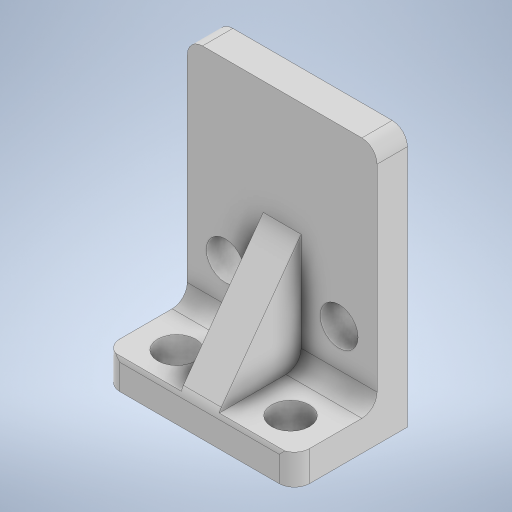
# Autodesk Inventor part: BP_L
Saved by Autodesk Inventor 2024.3 (Build 283343000, 343)
## iProperties
Created: 2025-10-31
Part Number: BP_L
Material: 一般
Document SubType Name: Modeling
Designer: 佐藤智貴
Density: 1 g/cm^3
Appearance: 既定
Author: 佐藤智貴
Autodesk Inventor part; units mm, degrees
ref_plane "YZ Plane" through (0, 0, 0) normal (1, 0, 0) x (0, 1, 0)
ref_plane "XZ Plane" through (0, 0, 0) normal (0, 1, 0) x (-1, 0, 0)
ref_plane "XY Plane" through (0, 0, 0) normal (0, 0, 1) x (1, 0, 0)
sketch "スケッチ1" plane through (0, 0, 0) normal (0, 0, 1) x (1, 0, 0)
  line L0 (0, 0) -> (25, 0)
  line L1 (25, 0) -> (25, 4)
  line L2 (25, 4) -> (0, 4)
  line L3 (0, 4) -> (0, 0)
  dimension "d0" = 4
  dimension "d1" = 25
  constraints: 8 end point, 2 parallel, 1 horizontal, 1 perpendicular
  measures "d0" distance of L0.end L1.end
  measures "d1" distance between parallel lines of L3 L1
extrude "押し出し1" add sketch "スケッチ1" along normal blind 18.9
sketch "スケッチ2" plane through (0, 4, 0) normal (0, 1, 0) x (1, 0, 0)
  line L0 (0, 0) -> (0, -18.9) projected
  line L1 (25, 0) -> (25, -18.9) projected
  line L2 (0, 0) -> (25, 0)
  line L3 (25, 0) -> (25, -8)
  line L4 (25, -8) -> (0, -8)
  line L5 (0, -8) -> (0, 0)
  point P0 (0, -8)
  dimension "d4" = 8
  constraints: 8 end point, 2 parallel, 1 horizontal, 1 perpendicular, 1 point on line
  measures "d4" distance between parallel lines of L2 L4
extrude "押し出し2" add sketch "スケッチ2" along normal blind 30
sketch "スケッチ3" plane through (0, 4, 18.9) normal (0, 1, 0) x (1, 0, 0)
  line L0 (0, 10.9) -> (25, 10.9) projected
  line L1 (25, 10.9) -> (25, 0) projected
  point P0 (0, 18.9)
  point P1 (5, 4.5)
  point P2 (20, 4.5)
  dimension "d7" = 15
  dimension "d8" = 6.4
  dimension "d9" = 6.4
  dimension "d10" = 5
  measures "d7" distance of point (20, 4.5) point (5, 4.5)
  measures "d8" distance from line of L0 point (5, 4.5)
  measures "d9" distance from line of L0 point (20, 4.5)
  measures "d10" distance from line of L1 point (20, 4.5)
hole "穴1" at (5, 4, 14.4) at (20, 4, 14.4) direction (0, -1, 0) diameter 5 end through all
sketch "スケッチ4" plane through (0, 4, 8) normal (0, 0, 1) x (1, 0, 0)
  line L0 (25, 0) -> (0, 0) projected
  line L1 (0, 0) -> (0, 30) projected
  point P0 (0, -4)
  point P1 (5, 7)
  point P2 (20, 7)
  dimension "d18" = 7
  dimension "d19" = 7
  dimension "d20" = 15
  dimension "d21" = 5
  measures "d18" distance from line of L0 point (20, 7)
  measures "d19" distance from line of L0 point (5, 7)
  measures "d20" distance of point (20, 7) point (5, 7)
  measures "d21" distance from line of L1 point (5, 7)
hole "穴2" at (5, 11, 8) at (20, 11, 8) direction (0, 0, -1) diameter 5 end through all
sketch "スケッチ7" plane through (0, 4, 18.9) normal (0, 1, 0) x (1, 0, 0)
  line L0 (25, 10.9) -> (0, 10.9) projected
  line L1 (25, 0) -> (0, 0) projected
  line L2 (10, 10.9) -> (15, 10.9)
  line L3 (15, 10.9) -> (15, 0)
  line L4 (15, 0) -> (10, 0)
  line L5 (10, 0) -> (10, 10.9)
  line L6 (25, 10.9) -> (25, 0) projected
  point P0 (0, 18.9)
  point P1 (10, 0)
  point P2 (15, 10.9)
  dimension "d36" = 5
  dimension "d37" = 10
  constraints: 8 end point, 2 parallel, 2 point on line, 1 horizontal, 1 perpendicular
  measures "d36" distance between parallel lines of L3 L5
  measures "d37" distance between parallel lines of L6 L3
extrude "押し出し5" add sketch "スケッチ7" along normal blind 15 contours L3 L1 L5 L0
sketch "スケッチ8" plane through (10, 4, 8) normal (-1, 0, 0) x (0, 0, 1)
  line L0 (10.9, 0) -> (0, 0) projected
  line L1 (10.9, 0) -> (10.9, 15) projected
  line L2 (0, 15) -> (10.9, 15) projected
  line L3 (0, 0) -> (0, 15) projected
  line L4 (10.9, 0) -> (0, 15)
  point P0 (-8, -4)
  constraints: 2 end point
extrude "押し出し6" cut sketch "スケッチ8" against normal blind 15 contours L4 L2 L1
fillet "フィレット1" radius 2 7 edges at (0, 34, 4) (25, 34, 4) (25, 2, 18.9) (0, 2, 18.9) (20, 4, 8) (5, 4, 8) (12.5, 4, 18.9)
sketch "スケッチ9" plane through (0, 0, 0) normal (0, 0, -1) x (-1, 0, 0)
  line L0 (-37.1274, 50.0053) -> (12.2795, 50.0053)
  line L1 (12.2795, 50.0053) -> (12.2795, -2.3527)
  line L2 (12.2795, -2.3527) -> (-37.1274, -2.3527)
  line L3 (-37.1274, -2.3527) -> (-37.1274, 50.0053)
  point P0 (0, 0)
  constraints: 8 end point, 2 parallel, 1 horizontal, 1 perpendicular
extrude "押し出し7" cut sketch "スケッチ9" against normal blind 4
equation "\"d9\" = d8"
equation "\"d19\" = d18"
